draw handle (Autodesk Fusion 360 design; units mm, degrees)
Autodesk Fusion 360 part; units mm, degrees
sketch "Sketch1" plane through (0, 0, 0) normal (0, 1, 0) x (1, 0, 0)
  line L0 (60, 0) -> (60, -30)
  line L1 (60, -15) -> (100, -15)
  line L2 (60, -15) -> (20, -15)
  circle A0 centre (20, -15) radius 1.8325
  circle A1 centre (100, -15) radius 1.8325
  line L3 (20, -15) -> (20, -5)
  line L4 (20, -15) -> (20, -25)
  line L5 (100, -15) -> (100, 0)
  line L6 (100, -15) -> (100, -30)
  line L7 (20, -25) -> (100, -25)
  line L8 (20, -5) -> (100, -5)
  line L9 (20, -15) -> (15, -15)
  line L10 (100, -15) -> (105, -15)
  line L11 (105, -15) -> (105, 0)
  line L12 (105, 0) -> (105, -30)
  line L13 (15, -15) -> (15, 0)
  line L14 (15, 0) -> (15, -30)
  line L15 (20, -5) -> (15, -5)
  line L16 (20, -25) -> (15, -25)
  line L17 (100, -25) -> (105, -25)
  line L18 (100, -5) -> (105, -5)
  line L19 (100, -15) -> (95, -15)
  line L20 (95, -15) -> (95, -7.4755)
  line L21 (95, -7.4755) -> (95, -25)
  line L22 (20, -15) -> (25, -15)
  line L23 (25, -15) -> (25, -5)
  line L24 (25, -15) -> (25, -25)
  line L25 (15, -25) -> (105, -25)
  line L26 (105, -25) -> (105, -5)
  line L27 (105, -5) -> (15, -5)
  line L28 (15, -5) -> (15, -25)
  line L29 (25, -25) -> (95, -25)
  line L30 (95, -25) -> (95, -5)
  line L31 (95, -5) -> (25, -5)
  line L32 (25, -5) -> (25, -25)
  circle A2 centre (20, -15) radius 4
  circle A3 centre (100, -15) radius 4
  dimension "d3" = 40
  dimension "d4" = 40
  dimension "d5" = 3.6649
  dimension "d6" = 3.6649
  dimension "d7" = 10
  dimension "d8" = 10
  dimension "d9" = 5
  dimension "d10" = 5
  dimension "d11" = 5
  dimension "d12" = 5
  dimension "d21" = 8
  dimension "d22" = 8
  constraint perpendicular L0 L1
  constraint perpendicular L0 L2
  constraint coincident L2.end A0.centre
  constraint coincident L1.end A1.centre
  constraint perpendicular L2 L3
  constraint perpendicular L2 L4
  constraint coincident L6 L7.end
  constraint perpendicular L6 L7
  constraint coincident L5 L8.end
  constraint perpendicular L5 L8
  constraint perpendicular L3 L9
  constraint coincident L13 L15.end
  constraint perpendicular L3 L15
  constraint coincident L14 L16.end
  constraint perpendicular L14 L16
  constraint coincident L12 L17.end
  constraint perpendicular L12 L17
  constraint coincident L11 L18.end
  constraint parallel L1 L19
  constraint coincident L7 L21.end
  constraint perpendicular L7 L21
  constraint perpendicular L21 L22
  constraint coincident L8 L23.end
  constraint perpendicular L8 L23
  constraint coincident L7 L24.end
  constraint perpendicular L7 L24
  constraint horizontal L25
  constraint vertical L26
  constraint horizontal L27
  constraint vertical L28
  constraint horizontal L29
  constraint vertical L30
  constraint horizontal L31
  constraint vertical L32
  constraint coincident L27 L30.end
  constraint concentric A0 A2
  constraint concentric A1 A3
  measures "d3" distance of L1.start L1.end
  measures "d4" distance of L1.start L2.end
  measures "d5" diameter of A0
  measures "d6" diameter of A1
  measures "d7" distance of L2.end L3.end
  measures "d8" distance of L2.end L4.end
  measures "d9" distance of L2.end L9.end
  measures "d10" distance of L1.end L10.end
  measures "d11" distance of L1.end L19.end
  measures "d12" distance of L2.end L22.end
  measures "d21" diameter of A2
  measures "d22" diameter of A3
extrude "Extrude1" add sketch "Sketch1" along normal blind 25
shell "Shell1" thickness 3 removed faces 1 at (83.3333, 25, 11.6667)
fillet "Fillet1" radius 5 2 edges at (15, 0, 15) (105, 0, 15)
extrude "Extrude2" add 1 faces at (46, 3, 12.6667) along direction (0, 1, 0) blind 2
extrude "Extrude3" add 1 faces at (46, 5, 12.6667) along direction (0, 1, 0) blind 3
sketch "Sketch2" plane through (0, 25, 0) normal (0, 1, 0) x (-1, 0, 0)
  line L0 (-100, 8) -> (-102, 8)
  line L1 (-102, 8) -> (-102, 22)
  line L2 (-102, 22) -> (-18, 22)
  line L3 (-18, 22) -> (-18, 8)
  line L4 (-18, 8) -> (-100, 8)
  line L5 (-100, 5) -> (-15, 5)
  line L6 (-15, 5) -> (-15, 25)
  line L7 (-15, 25) -> (-105, 25)
  line L8 (-105, 25) -> (-105, 5)
  line L9 (-105, 5) -> (-100, 5)
  circle A0 centre (-100, 15) radius 4
  circle A1 centre (-20, 15) radius 4
  circle A2 centre (-20, 15) radius 1.8324
  circle A3 centre (-100, 15) radius 1.8325
  point P0 (-100, 15)
  point P1 (-20, 15)
  constraint coincident P0 A0.centre
  constraint coincident P1 A1.centre
extrude "Extrude4" add sketch "Sketch2" against normal blind 19 contours L1 A0 | L1 A0 | L3 A1 | L3 A1
sketch "Sketch3" plane through (0, 0, 8) normal (0, 0, 1) x (1, 0, 0)
  line L0 (18, 8) -> (100, 8)
  line L1 (100, 8) -> (100, 25)
  line L2 (100, 25) -> (18, 25)
  line L3 (18, 25) -> (18, 8)
  line L4 (18, 25) -> (23, 25)
  line L5 (23, 25) -> (23, 9)
  line L6 (23, 9) -> (26, 9)
  line L7 (26, 9) -> (26, 25)
  line L8 (102, 25) -> (97, 25)
  line L9 (97, 25) -> (97, 9)
  line L10 (97, 9) -> (94, 9)
  line L11 (94, 9) -> (94, 25)
  dimension "d25" = 3
  dimension "d26" = 5
  dimension "d27" = 3
  constraint coincident L2.end L3.start
  constraint coincident L2 L4.end
  constraint perpendicular L3 L4
  constraint perpendicular L0 L5
  constraint perpendicular L3 L6
  constraint coincident L2 L7.end
  constraint perpendicular L2 L7
  constraint parallel L2 L8
  constraint perpendicular L8 L9
  constraint perpendicular L9 L10
  constraint vertical L11
  constraint coincident L2 L11.end
  measures "d25" distance of L5.end L6.end
  measures "d26" distance of L8.start L8.end
  measures "d27" distance of L9.end L10.end
extrude "Extrude5" add sketch "Sketch3" along normal blind 16 contours L2 L5 L6 L7 | L2 L9 L10 L11
sketch "Sketch4" plane through (0, 0, 8) normal (0, 0, 1) x (1, 0, 0)
  line L0 (23, 9) -> (23, 25)
  line L1 (23, 25) -> (18, 25)
  line L2 (18, 25) -> (18, 8)
  line L3 (18, 8) -> (100, 8)
  line L4 (100, 8) -> (100, 25)
  line L5 (100, 25) -> (97, 25)
  line L6 (97, 25) -> (97, 9)
  line L7 (97, 9) -> (94, 9)
  line L8 (94, 9) -> (94, 25)
  line L9 (94, 25) -> (26, 25)
  line L10 (26, 25) -> (26, 9)
  line L11 (26, 9) -> (23, 9)
  line L12 (26.0298, 8) -> (26, 8)
  line L13 (26, 8) -> (26, 25)
  line L14 (26, 25) -> (26.0298, 25)
  line L15 (26.0298, 25) -> (26.0298, 8)
  line L16 (26, 8) -> (94, 8)
  line L17 (94, 8) -> (94, 25)
  line L18 (94, 25) -> (26, 25)
  line L19 (26, 25) -> (26, 8)
  constraint horizontal L12
  constraint vertical L13
  constraint horizontal L14
  constraint vertical L15
  constraint coincident L9.end L10.start
  constraint coincident L3 L12.start
  constraint horizontal L16
  constraint vertical L17
  constraint horizontal L18
  constraint vertical L19
  constraint coincident L8.end L9.start
extrude "Extrude6" add 1 faces at (103.9442, 25, 15) along direction (0, -1, 0) blind 17
extrude "Extrude7" cut sketch "Sketch4" along normal mid plane 50 contours L3 L8 L9 L15 L16 L17 L18
fillet "Fillet2" radius 5 4 edges at (94, 8, 15) (26, 8, 15) (26.0298, 8, 23.5) (26.0298, 8, 6.5)
fillet "Fillet3" radius 3 2 edges at (101.7084, 25, 15.6626) (21.7084, 25, 15.6626)
chamfer "Chamfer1" distance 2 angle 45 10 edges at (26.0298, 19, 5) (27.4943, 9.4645, 5) (60.0149, 8, 5) (92.5355, 9.4645, 5) (94, 19, 5) (94, 19, 25) (92.5355, 9.4645, 25) (60.0149, 8, 25) (27.4943, 9.4645, 25) (26.0298, 19, 25)
chamfer "Chamfer2" distance 2 angle 45 10 edges at (105, 15, 5) (103.5355, 1.4645, 5) (60, 0, 5) (16.4645, 1.4645, 5) (15, 15, 5) (105, 15, 25) (103.5355, 1.4645, 25) (60, 0, 25) (16.4645, 1.4645, 25) (15, 15, 25)
